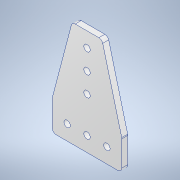
# Autodesk Inventor part: プレート保持_固定具1
Saved by Autodesk Inventor 2021 (Build 250183000, 183)
## iProperties
Created: 2022-02-03
Part Number: プレート保持_固定具1
Material: アルミニウム 6061
Document SubType Name: Modeling
Designer: hirohumi
Density: 2.7 g/cm^3
Appearance: アルミニウム - フラット
Author: hirohumi
Autodesk Inventor part; units mm, degrees
ref_plane "YZ Plane" through (0, 0, 0) normal (1, 0, 0) x (0, 1, 0)
ref_plane "XZ Plane" through (0, 0, 0) normal (0, 1, 0) x (-1, 0, 0)
ref_plane "XY Plane" through (0, 0, 0) normal (0, 0, 1) x (1, 0, 0)
sketch "スケッチ1" plane through (0, 0, 0) normal (0, 0, 1) x (1, 0, 0)
  circle A0 centre (0, 0) radius 1.6
  circle A1 centre (10, 0) radius 1.6
  circle A2 centre (-10, 0) radius 1.6
  circle A3 centre (0, 18) radius 1.6
  circle A4 centre (0, 28) radius 1.6
  circle A5 centre (0, 38) radius 1.6
  line L0 (-7.5, 45.5) -> (7.5, 45.5)
  line L1 (7.5, 45.5) -> (17.5, 7.5)
  line L2 (17.5, 7.5) -> (17.5, -7.5)
  line L3 (17.5, -7.5) -> (-17.5, -7.5)
  line L4 (-17.5, -7.5) -> (-17.5, 7.5)
  line L5 (-17.5, 7.5) -> (-7.5, 45.5)
  dimension "d0" = 3.2
  dimension "d1" = 3.2
  dimension "d2" = 3.2
  dimension "d3" = 10
  dimension "d4" = 10
  dimension "d5" = 3.2
  dimension "d6" = 3.2
  dimension "d7" = 3.2
  dimension "d8" = 10
  dimension "d9" = 10
  dimension "d10" = 18
  dimension "d11" = 7.5
  dimension "d13" = 7.5
  dimension "d14" = 7.5
  dimension "d15" = 7.5
  dimension "d16" = 7.5
  dimension "d17" = 7.5
  dimension "d18" = 7.5
  dimension "d19" = 7.5
  constraints: 12 end point, 6 centre point, 3 perpendicular, 3 vertical alignment, 2 horizontal alignment, 1 coincident, 1 horizontal
  measures "d0" diameter of A0
  measures "d1" diameter of A1
  measures "d2" diameter of A2
  measures "d3" distance of point (0, 0) A2.centre
  measures "d4" distance of A1.centre point (0, 0)
  measures "d5" diameter of A3
  measures "d6" diameter of A4
  measures "d7" diameter of A5
  measures "d8" distance of A4.centre A3.centre
  measures "d9" distance of A5.centre A4.centre
  measures "d10" distance of point (0, 0) A3.centre
  measures "d11" distance from line of A5.centre L0
  measures "d13" distance from line of L3 A2.centre
  measures "d14" distance from line of A2.centre L4
  measures "d15" distance from line of L2 A1.centre
  measures "d16" horizontal distance of A5.centre L0.start
  measures "d17" horizontal distance of A5.centre L0.end
  measures "d18" horizontal distance of A2.centre L4.end
  measures "d19" horizontal distance of A1.centre L1.end
extrude "押し出し1" add sketch "スケッチ1" along normal blind 3
fillet "フィレット1" radius 2 6 edges at (-7.5, 45.5, 1.5) (7.5, 45.5, 1.5) (17.5, 7.5, 1.5) (17.5, -7.5, 1.5) (-17.5, -7.5, 1.5) (-17.5, 7.5, 1.5)
